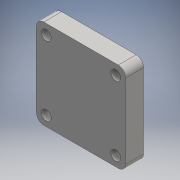
# Autodesk Inventor part: Bearing_Block
Saved by Autodesk Inventor 2016 (Build 200138000, 138)
## iProperties
Created: 2016-04-11
Part Number: Bearing_Block
Material: Generic
Document SubType Name: Modeling
Designer: agmle
Density: 1 g/cm^3
Appearance: Default
Author: agmle
Autodesk Inventor part; units mm, degrees
ref_plane "YZ Plane" through (0, 0, 0) normal (1, 0, 0) x (0, 1, 0)
ref_plane "XZ Plane" through (0, 0, 0) normal (0, 1, 0) x (-1, 0, 0)
ref_plane "XY Plane" through (0, 0, 0) normal (0, 0, 1) x (1, 0, 0)
sketch "Sketch1" plane through (0, 0, 0) normal (0, 1, 0) x (-1, 0, 0)
  line L0 (16.6369, 20.0223) -> (-15.1131, 20.0223)
  line L1 (-18.2881, 16.8473) -> (-18.2881, -14.9027)
  line L2 (-15.1131, -18.0777) -> (16.6369, -18.0777)
  line L3 (19.8119, -14.9027) -> (19.8119, 16.8473)
  arc A0 (19.8119, 16.8473) -> (16.6369, 20.0223) centre (16.6369, 16.8473) ccw
  arc A1 (-18.2881, -14.9027) -> (-15.1131, -18.0777) centre (-15.1131, -14.9027) ccw
  arc A2 (16.6369, -18.0777) -> (19.8119, -14.9027) centre (16.6369, -14.9027) ccw
  arc A3 (-15.1131, 20.0223) -> (-18.2881, 16.8473) centre (-15.1131, 16.8473) ccw
  point P0 (0, 0)
  dimension "d0" = 38.1
  dimension "d1" = 3.175
  constraints: 8 end point, 8 point on circle, 8 tangent, 4 centre point, 3 equal radius, 2 parallel, 2 perpendicular, 1 horizontal
  measures "d0" distance between parallel lines of L2 L0
  measures "d1" radius of A0
extrude "Extrusion1" add sketch "Sketch1" along normal blind 7.62
sketch "Sketch2" plane through (0, 7.62, 0) normal (0, 1, 0) x (1, 0, 0)
  line L0 (-19.8119, 14.9027) -> (-19.8119, -16.8473) projected
  line L1 (-16.6369, -20.0223) -> (15.1131, -20.0223) projected
  line L2 (15.1131, 18.0777) -> (-16.6369, 18.0777) projected
  line L3 (18.2881, -16.8473) -> (18.2881, 14.9027) projected
  point P0 (0, 0)
  point P1 (-15.5619, -15.7723)
  point P2 (-15.5619, 13.8277)
  point P3 (14.0381, 13.8277)
  point P4 (14.0381, -15.7723)
  dimension "d4" = 4.25
  dimension "d5" = 4.25
  dimension "d6" = 4.25
  dimension "d7" = 4.25
  dimension "d8" = 4.25
  dimension "d9" = 4.25
  dimension "d10" = 4.25
  dimension "d11" = 4.25
  measures "d4" distance from line of L0 point (-15.562, -15.772)
  measures "d5" distance from line of L1 point (-15.562, -15.772)
  measures "d6" distance from line of L0 point (-15.562, 13.828)
  measures "d7" distance from line of L2 point (-15.562, 13.828)
  measures "d8" distance from line of L2 point (14.038, 13.828)
  measures "d9" distance from line of L3 point (14.038, 13.828)
  measures "d10" distance from line of L3 point (14.038, -15.772)
  measures "d11" distance from line of L1 point (14.038, -15.772)
hole "Hole1" at (-15.5619, 7.62, 15.7723) at (-15.5619, 7.62, -13.8277) at (14.0381, 7.62, -13.8277) at (14.0381, 7.62, 15.7723) direction (0, -1, 0) diameter 4.2 end through all
equation "\"d5\" = d4"
equation "\"d6\" = d4"
equation "\"d7\" = d4"
equation "\"d8\" = d4"
equation "\"d9\" = d4"
equation "\"d10\" = d4"
equation "\"d11\" = d4"
body "Solid1"
